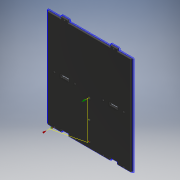
# Autodesk Inventor part: BA04
Saved by Autodesk Inventor 2017 (Build 210142000, 142)
## iProperties
Created: 2019-05-22
Part Number: BA04
Material: Polyethylene, High Density
Document SubType Name: Modeling
Designer: Dell
Density: 0.952 g/cm^3
Appearance: Smooth - Black
Mass: 627.857 g
Surface Area: 2193.54 cm^2
Volume: 659.513 cm^3
Author: Dell
Autodesk Inventor part; units mm, degrees
ref_plane "YZ Plane" through (0, 0, 0) normal (1, 0, 0) x (0, 1, 0)
ref_plane "XZ Plane" through (0, 0, 0) normal (0, 1, 0) x (-1, 0, 0)
ref_plane "XY Plane" through (0, 0, 0) normal (0, 0, 1) x (1, 0, 0)
sketch "Sketch1" plane through (0, 0, 0) normal (0, 0, 1) x (1, 0, 0)
  line L0 (0, 0) -> (303.5592, 0)
  line L1 (303.5592, 0) -> (455.3388, -262.89) construction
  line L2 (455.3388, -262.89) -> (404.5388, -350.8782)
  line L3 (404.5388, -350.8782) -> (-50.8, -87.9882) construction
  line L4 (-50.8, -87.9882) -> (0, 0) construction
  line L5 (0, 0) -> (3.6662, -6.35)
  line L6 (3.6662, -6.35) -> (299.8931, -6.35)
  line L7 (299.8931, -6.35) -> (303.5592, 0)
  dimension "d0" = 525.78
  dimension "d1" = 101.6
  dimension "d2" = 120
  dimension "d3" = 6.35
  dimension "d4" = 60
  dimension "d5" = 60
  constraints: 16 end point, 2 equal length, 2 horizontal, 2 perpendicular
  measures "d0" distance of L2.end L3.end
  measures "d1" distance of L3.end L0.start
  measures "d2" angle of L0 L4
  measures "d3" distance between parallel lines of L0 L6
  measures "d4" angle of L0 L5
  measures "d5" angle of L0 L7
extrude "Extrusion1" add sketch "Sketch1" along normal blind 349.25
sketch "Sketch2" plane through (3.6662, -6.35, 0) normal (0, -1, 0) x (1, 0, 0)
  line L0 (299.8931, 349.25) -> (-3.6662, 349.25) projected
  line L1 (47.1338, 349.25) -> (72.5338, 349.25)
  line L2 (72.5338, 349.25) -> (72.5338, 355.6)
  line L3 (72.5338, 355.6) -> (47.1338, 355.6)
  line L4 (47.1338, 355.6) -> (47.1338, 349.25)
  line L5 (223.6931, 349.25) -> (249.0931, 349.25)
  line L6 (249.0931, 349.25) -> (249.0931, 355.6)
  line L7 (249.0931, 355.6) -> (223.6931, 355.6)
  line L8 (223.6931, 355.6) -> (223.6931, 349.25)
  line L9 (-3.6662, 0) -> (-3.6662, 349.25) projected
  line L10 (299.8931, 0) -> (299.8931, 349.25) projected
  circle A0 centre (59.8338, 352.425) radius 2.25
  circle A1 centre (236.3931, 352.425) radius 2.25
  point P0 (59.8338, 355.6)
  point P1 (236.3931, 355.6)
  point P2 (72.5338, 352.425)
  point P3 (249.0931, 352.425)
  dimension "d8" = 25.4
  dimension "d9" = 6.35
  dimension "d10" = 25.4
  dimension "d11" = 6.35
  dimension "d12" = 50.8
  dimension "d13" = 50.8
  dimension "d16" = 4.5
  dimension "d17" = 4.5
  constraints: 16 end point, 4 midpoint, 4 parallel, 2 centre point, 2 horizontal, 2 horizontal alignment, 2 perpendicular, 2 point on line, 2 vertical alignment
  measures "d8" distance of L3.end L2.end
  measures "d9" distance of L2.end L1.end
  measures "d10" distance of L7.end L6.end
  measures "d11" distance of L6.end L5.end
  measures "d12" distance between parallel lines of L9 L4
  measures "d13" distance between parallel lines of L10 L6
  measures "d16" diameter of A0
  measures "d17" diameter of A1
extrude "Extrusion2" add sketch "Sketch2" against normal blind 6.35
ref_plane "Work Plane1" through (0, 0, 298.45) normal (0, 0, 1) x (1, 0, 0)
sketch "Sketch3" plane through (0, 0, 298.45) normal (0, 0, 1) x (1, 0, 0)
  line L0 (0, 0) -> (303.5592, 0) projected
  line L1 (0, 0) -> (0, -6.35)
  line L2 (299.8931, -6.35) -> (3.6662, -6.35) projected
  line L3 (0, -6.35) -> (3.6662, -6.35)
  line L4 (3.6662, -6.35) -> (0, 0) projected
  constraints: 4 end point, 1 perpendicular, 1 vertical
extrude "Extrusion3" [suppressed]
ref_plane "Work Plane2" through (0, 0, 50.8) normal (0, 0, -1) x (-1, 0, 0)
sketch "Sketch4" plane through (0, 0, 50.8) normal (0, 0, -1) x (-1, 0, 0)
  line L0 (0, -12.7) -> (0, 0) projected
  line L1 (-7.3323, -12.7) -> (0, 0) projected
  line L2 (-7.3323, -12.7) -> (0, -12.7) projected
extrude "Extrusion4" [suppressed]
ref_plane "Work Plane3" through (0, 0, 174.625) normal (0, 0, -1) x (-1, 0, 0)
sketch "Sketch5" plane through (0, 0, 174.625) normal (0, 0, -1) x (-1, 0, 0)
  line L0 (0, 0) -> (0, -12.7) projected
  line L1 (0, -12.7) -> (-7.3323, -12.7) projected
  line L2 (0, 0) -> (-7.3323, -12.7) projected
extrude "Extrusion5" [suppressed]
ref_plane "Work Plane4" through (151.7796, -6.35, 349.25) normal (-1, 0, 0) x (0, 0, 1)
mirror "Mirror1" [suppressed]
sketch "Sketch6" plane through (296.2269, -12.7, 292.1) normal (0, 0, 1) x (1, 0, 0)
  line L0 (0, 0) -> (7.3323, 12.7) projected
  line L1 (7.3323, 0) -> (0, 0) projected
  line L2 (7.3323, 12.7) -> (7.3323, 0) projected
  line L3 (7.3323, 12.7) -> (7.3323, 0) projected
  line L4 (0, 0) -> (7.3323, 12.7) projected
  line L5 (7.3323, 0) -> (0, 0) projected
  line L6 (-296.2269, 12.7) -> (-296.2269, 0) projected
  line L7 (-296.2269, 0) -> (-288.8945, 0) projected
  line L8 (-296.2269, 12.7) -> (-288.8945, 0) projected
  line L9 (-296.2269, 0) -> (-296.2269, 12.7) projected
  line L10 (-296.2269, 12.7) -> (-274.2298, 0) construction
  line L11 (0, 0) -> (-288.8945, 0) projected
  line L12 (-285.2269, 6.3491) -> (-285.2269, 0)
  line L13 (-288.8945, 0) -> (-296.2269, 0) projected
  line L14 (-285.2269, 0) -> (-296.2269, 0)
  line L15 (-144.4473, 0) -> (-144.4473, -42.8761)
  line L16 (7.3323, 12.7) -> (7.3323, 0)
  line L17 (7.3323, 0) -> (0, 0)
  line L18 (7.3323, 12.7) -> (0, 0)
  line L19 (7.3323, 0) -> (7.3323, 12.7)
  line L20 (7.3323, 12.7) -> (-14.6647, 0) construction
  line L21 (-3.6677, 6.3491) -> (-3.6677, 0)
  line L22 (0, 0) -> (7.3323, 0)
  line L23 (-3.6677, 0) -> (7.3323, 0)
  line L24 (-288.8945, 0) -> (-296.2269, 12.7) projected
  line L25 (-285.2269, 6.3491) -> (-296.2269, 12.7)
  line L26 (7.3323, 12.7) -> (0, 0) projected
  line L27 (7.3323, 12.7) -> (-3.6677, 6.3491)
  line L28 (0, 0) -> (7.3323, 12.7)
  line L29 (0, 0) -> (-3.6677, 0)
  line L30 (7.3323, 0) -> (7.3323, 12.7) projected
  line L31 (-3.6677, 0) -> (7.3323, 0)
  dimension "d26" = 60
  dimension "d27" = 11
  constraints: 34 end point, 5 symmetric about line, 3 point on line, 2 collinear, 2 horizontal, 1 midpoint, 1 perpendicular, 1 vertical
  measures "d26" angle of L6 L10
  measures "d27" distance between parallel lines of L6 L12
extrude "Extrusion6" [suppressed]
sketch "Sketch7" plane through (0, 0, 184.15) normal (0, 0, 1) x (1, 0, 0)
  line L0 (7.3323, -12.7) -> (0, 0) projected
  line L1 (11, -12.7) -> (7.3323, -12.7) projected
  line L2 (11, -6.3509) -> (11, -12.7) projected
  line L3 (0, 0) -> (11, -6.3509) projected
  line L4 (303.5592, 0) -> (296.2269, -12.7) projected
  line L5 (292.5592, -6.3509) -> (303.5592, 0) projected
  line L6 (292.5592, -12.7) -> (292.5592, -6.3509) projected
  line L7 (296.2269, -12.7) -> (292.5592, -12.7) projected
  line L8 (303.5592, 0) -> (303.5592, -12.7) projected
  line L9 (296.2269, -12.7) -> (303.5592, 0) projected
  line L10 (303.5592, -12.7) -> (296.2269, -12.7) projected
  line L11 (0, 0) -> (0, -12.7) projected
  line L12 (0, -12.7) -> (7.3323, -12.7) projected
  line L13 (0, 0) -> (7.3323, -12.7) projected
extrude "Extrusion7" [suppressed]
sketch "Sketch8" plane through (0, 0, 76.2) normal (0, 0, 1) x (1, 0, 0)
  line L0 (0, 0) -> (0, -12.7) projected
  line L1 (0, -12.7) -> (7.3323, -12.7) projected
  line L2 (0, 0) -> (7.3323, -12.7) projected
  line L3 (7.3323, -12.7) -> (0, 0) projected
  line L4 (11, -12.7) -> (7.3323, -12.7) projected
  line L5 (11, -6.3509) -> (11, -12.7) projected
  line L6 (0, 0) -> (11, -6.3509) projected
  line L7 (303.5592, 0) -> (296.2269, -12.7) projected
  line L8 (292.5592, -6.3509) -> (303.5592, 0) projected
  line L9 (292.5592, -12.7) -> (292.5592, -6.3509) projected
  line L10 (296.2269, -12.7) -> (292.5592, -12.7) projected
  line L11 (303.5592, 0) -> (303.5592, -12.7) projected
  line L12 (296.2269, -12.7) -> (303.5592, 0) projected
  line L13 (303.5592, -12.7) -> (296.2269, -12.7) projected
extrude "Extrusion8" [suppressed]
sketch "Sketch9" plane through (0, 0, 0) normal (0, 0, -1) x (-1, 0, 0)
  line L0 (-251.9796, -6.35) -> (-251.9796, 0)
  line L1 (-251.9796, 0) -> (-226.5796, 0)
  line L2 (-226.5796, 0) -> (-226.5796, -6.35)
  line L3 (-226.5796, -6.35) -> (-251.9796, -6.35)
  line L4 (-76.9796, -6.35) -> (-76.9796, 0)
  line L5 (-76.9796, 0) -> (-51.5796, 0)
  line L6 (-51.5796, 0) -> (-51.5796, -6.35)
  line L7 (-51.5796, -6.35) -> (-76.9796, -6.35)
  line L8 (-239.2796, 0) -> (-64.2796, 0) construction
  circle A0 centre (-239.2796, -3.175) radius 2.25
  circle A1 centre (-64.2796, -3.175) radius 2.25
  line L9 (-239.2796, -3.175) -> (-239.2796, 0) construction
  line L10 (-239.2796, -3.175) -> (-226.5796, -3.175) construction
  line L11 (-76.9796, -3.175) -> (-64.2796, -3.175) construction
  line L12 (-64.2796, -3.175) -> (-64.2796, 0) construction
  line L13 (0, 0) -> (-303.5592, 0) projected
  point P0 (-151.7796, 0)
  dimension "d34" = 25.4
  dimension "d35" = 6.35
  dimension "d36" = 6.35
  dimension "d37" = 25.4
  dimension "d38" = 175
  dimension "d39" = 4.5
  dimension "d40" = 4.5
  constraints: 26 end point, 6 midpoint, 6 perpendicular, 4 parallel, 4 point on line, 2 centre point
  measures "d34" distance of L4.end L5.end
  measures "d35" distance of L5.end L7.start
  measures "d36" distance of L0.start L1.start
  measures "d37" distance of L1.start L2.start
  measures "d38" distance of L8.start L12.end
  measures "d39" diameter of A0
  measures "d40" diameter of A1
extrude "Extrusion9" cut sketch "Sketch9" against normal blind 6.35 contours L0 L1 L2 L3 | L4 L5 L6 L7 | A0 | A1
sketch "Sketch10" plane through (227.3592, -6.35, 355.6) normal (0, -1, 0) x (1, 0, 0)
  line L0 (-175.7796, -184.625) -> (-150.3796, -184.625)
  line L1 (-150.3796, -184.625) -> (-150.3796, -178.275)
  line L2 (-150.3796, -178.275) -> (-175.7796, -178.275)
  line L3 (-175.7796, -178.275) -> (-175.7796, -184.625)
  line L4 (-0.7796, -184.625) -> (24.6204, -184.625)
  line L5 (24.6204, -184.625) -> (24.6204, -178.275)
  line L6 (24.6204, -178.275) -> (-0.7796, -178.275)
  line L7 (-0.7796, -178.275) -> (-0.7796, -184.625)
  line L8 (-175.7796, -349.25) -> (-150.3796, -349.25) projected
  line L9 (-0.7796, -349.25) -> (24.6204, -349.25) projected
  line L10 (76.2, -6.35) -> (-227.3592, -6.35) projected
  point P0 (-227.3592, -355.6)
  point P1 (-163.0796, -184.625)
  point P2 (-163.0796, -349.25)
  point P3 (11.9204, -184.625)
  point P4 (11.9204, -349.25)
  point P5 (-176.5592, -6.35)
  dimension "d44" = 25.4
  dimension "d45" = 6.35
  dimension "d46" = 25.4
  dimension "d47" = 6.35
  dimension "d90" = 171.925
  constraints: 16 end point, 4 midpoint, 4 parallel, 2 horizontal, 2 perpendicular, 2 vertical alignment, 1 horizontal alignment
  measures "d44" distance of L2.end L1.end
  measures "d45" distance of L1.end L0.end
  measures "d46" distance of L6.end L5.end
  measures "d47" distance of L5.end L4.end
  measures "d90" distance between parallel lines of L10 L2
extrude "Extrusion10" cut sketch "Sketch10" against normal through all
sketch "Sketch11" plane through (227.3592, -6.35, 355.6) normal (0, -1, 0) x (1, 0, 0)
  line L0 (-150.3796, -355.6) -> (-0.7796, -355.6) construction
  line L1 (-100.9796, -355.6) -> (-50.1796, -355.6) construction
  line L2 (-50.1796, -355.6) -> (-50.1796, -178.275) construction
  line L3 (-50.1796, -178.275) -> (-100.9796, -178.275) construction
  line L4 (-100.9796, -178.275) -> (-100.9796, -355.6) construction
  circle A0 centre (-75.5796, -267.89) radius 4
  circle A1 centre (-75.5796, -200.18) radius 4
  circle A2 centre (-75.5796, -335.6) radius 4
  line L5 (-0.7796, -355.6) -> (-150.3796, -355.6) projected
  circle A3 centre (-199.7363, -181.45) radius 2.25
  circle A4 centre (-199.7363, -352.425) radius 2.25
  circle A5 centre (48.5771, -352.425) radius 2.25
  circle A6 centre (48.5771, -181.45) radius 2.25
  line L6 (-175.7796, -355.6) -> (-223.6931, -355.6) projected
  line L7 (72.5338, -355.6) -> (24.6204, -355.6) projected
  line L8 (-175.7796, -184.625) -> (-175.7796, -178.275) projected
  line L9 (-175.7796, -355.6) -> (-175.7796, -349.25) projected
  line L10 (24.6204, -349.25) -> (24.6204, -355.6) projected
  line L11 (24.6204, -178.275) -> (24.6204, -184.625) projected
  circle A7 centre (-126.3796, -181.45) radius 2.25
  circle A8 centre (-126.3796, -352.425) radius 2.25
  circle A9 centre (-24.7796, -352.425) radius 2.25
  circle A10 centre (-24.7796, -181.45) radius 2.25
  point P0 (-227.3592, -355.6)
  point P1 (-150.3796, -178.275)
  point P2 (-75.5796, -355.6)
  point P3 (-75.5796, -355.6)
  point P4 (-75.5796, -355.6)
  point P5 (-50.1796, -266.9375)
  point P6 (-199.7363, -355.6)
  point P7 (48.5771, -355.6)
  point P8 (-175.7796, -181.45)
  point P9 (-175.7796, -352.425)
  point P10 (24.6204, -352.425)
  point P11 (24.6204, -181.45)
  point P12 (24.6204, -352.425)
  dimension "d52" = 8
  dimension "d53" = 8
  dimension "d54" = 8
  dimension "d56" = 20
  dimension "d59" = 50.8
  dimension "d60" = 4.5
  dimension "d61" = 4.5
  dimension "d62" = 4.5
  dimension "d63" = 4.5
  dimension "d64" = 4.5
  dimension "d65" = 4.5
  dimension "d66" = 4.5
  dimension "d67" = 4.5
  dimension "d68" = 25.4
  dimension "d69" = 25.4
  dimension "d96" = 67.71
  dimension "d97" = 67.71
  constraints: 11 centre point, 11 midpoint, 9 horizontal alignment, 9 vertical alignment, 8 end point, 2 parallel, 1 coincident, 1 horizontal, 1 perpendicular, 1 point on line
  measures "d52" diameter of A0
  measures "d53" diameter of A1
  measures "d54" diameter of A2
  measures "d56" distance from line of L0 A2.centre
  measures "d59" distance of L2.end L3.end
  measures "d60" diameter of A3
  measures "d61" diameter of A4
  measures "d62" diameter of A5
  measures "d63" diameter of A6
  measures "d64" diameter of A7
  measures "d65" diameter of A8
  measures "d66" diameter of A9
  measures "d67" diameter of A10
  measures "d68" distance from line of L2 A10.centre
  measures "d69" distance from line of A7.centre L4
  measures "d96" distance of A0.centre A1.centre
  measures "d97" distance of A2.centre A0.centre
extrude "Extrusion11" cut sketch "Sketch11" against normal through all
sketch "Sketch12" plane through (227.3592, -6.35, 355.6) normal (0, -1, 0) x (1, 0, 0)
  line L0 (-175.7796, -355.6) -> (-223.6931, -355.6) projected
  line L1 (-177.0496, -355.6) -> (-149.1096, -355.6)
  line L2 (-149.1096, -355.6) -> (-149.1096, -347.98)
  line L3 (-149.1096, -347.98) -> (-177.0496, -347.98)
  line L4 (-177.0496, -347.98) -> (-177.0496, -355.6)
  line L5 (-0.7796, -355.6) -> (-150.3796, -355.6) projected
  line L6 (-2.0496, -355.6) -> (25.8904, -355.6)
  line L7 (25.8904, -355.6) -> (25.8904, -347.98)
  line L8 (25.8904, -347.98) -> (-2.0496, -347.98)
  line L9 (-2.0496, -347.98) -> (-2.0496, -355.6)
  line L10 (-177.0496, -177.005) -> (-149.1096, -177.005)
  line L11 (-149.1096, -177.005) -> (-149.1096, -185.895)
  line L12 (-149.1096, -185.895) -> (-177.0496, -185.895)
  line L13 (-177.0496, -185.895) -> (-177.0496, -177.005)
  line L14 (-2.0496, -177.005) -> (25.8904, -177.005)
  line L15 (25.8904, -177.005) -> (25.8904, -185.895)
  line L16 (25.8904, -185.895) -> (-2.0496, -185.895)
  line L17 (-2.0496, -185.895) -> (-2.0496, -177.005)
  line L18 (-150.3796, -178.275) -> (-150.3796, -184.625) projected
  line L19 (-0.7796, -184.625) -> (-0.7796, -178.275) projected
  line L20 (-175.7796, -178.275) -> (-150.3796, -178.275) projected
  line L21 (-0.7796, -178.275) -> (24.6204, -178.275) projected
  line L22 (-0.7796, -349.25) -> (24.6204, -349.25) projected
  line L23 (-175.7796, -349.25) -> (-150.3796, -349.25) projected
  circle A0 centre (-178.8043, -4.1049) radius 3.175
  circle A1 centre (-148.9142, -4.1049) radius 3.175
  circle A2 centre (-2.2451, -4.1049) radius 3.175
  circle A3 centre (27.6451, -4.1049) radius 3.175
  line L24 (-176.5592, -6.35) -> (-178.8043, -4.1049)
  line L25 (-223.6931, -6.35) -> (-176.5592, -6.35) projected
  point P0 (-227.3592, -355.6)
  point P1 (-150.3796, -181.45)
  point P2 (-149.1096, -181.45)
  point P3 (-0.7796, -181.45)
  point P4 (-2.0496, -181.45)
  point P5 (-163.0796, -178.275)
  point P6 (-163.0796, -177.005)
  point P7 (11.9204, -178.275)
  point P8 (11.9204, -177.005)
  point P9 (11.9204, -349.25)
  point P10 (11.9204, -347.98)
  point P11 (-163.0796, -349.25)
  point P12 (-163.0796, -347.98)
  point P13 (-151.1592, -6.35)
  point P14 (0, -6.35)
  point P15 (25.4, -6.35)
  dimension "d74" = 6.35
  dimension "d75" = 6.35
  dimension "d76" = 6.35
  dimension "d77" = 6.35
  dimension "d70" = 1.27
  dimension "d71" = 1.27
  dimension "d72" = 1.27
  dimension "d73" = 1.27
  dimension "d89" = 45
  constraints: 34 end point, 12 midpoint, 8 parallel, 7 horizontal alignment, 5 vertical alignment, 4 horizontal, 4 perpendicular, 3 point on line, 12 other
  measures "d70" distance between parallel lines of L10 L20
  measures "d71" distance between parallel lines of L17 L19
  measures "d72" distance between parallel lines of L11 L18
  measures "d73" distance between parallel lines of L3 L23
  measures "d89" angle of L25 L24
extrude "Extrusion12" cut sketch "Sketch12" against normal through all
sketch "Sketch13" plane through (227.3592, -6.35, 355.6) normal (0, -1, 0) x (1, 0, 0)
  line L0 (-176.5592, 0) -> (-151.1592, 0)
  line L1 (-151.1592, 0) -> (-151.1592, 1.27)
  line L2 (-151.1592, 1.27) -> (-176.5592, 1.27)
  line L3 (-176.5592, 1.27) -> (-176.5592, 0)
  line L4 (25.4, 0) -> (0, 0)
  line L5 (0, 0) -> (0, 1.27)
  line L6 (0, 1.27) -> (25.4, 1.27)
  line L7 (25.4, 1.27) -> (25.4, 0)
  point P0 (-227.3592, -355.6)
  point P1 (-151.1592, 0)
  dimension "d80" = 1.27
  constraints: 16 end point, 4 parallel, 2 coincident, 2 horizontal, 2 perpendicular, 1 horizontal alignment
  measures "d80" distance of L2.end L0.start
extrude "Extrusion13" add sketch "Sketch13" against normal up to surface (6.35 mm away) from surface at 0
sketch "Sketch14" plane through (299.8931, -6.35, 0) normal (0, -1, 0) x (1, 0, 0)
  line L0 (-47.1338, 356.87) -> (-72.5338, 356.87) projected
  line L1 (-47.1338, 356.87) -> (-47.7688, 356.87)
  line L2 (-47.7688, 356.87) -> (-47.7688, 352.8314)
  line L3 (-47.7688, 352.8314) -> (-47.1338, 352.8314)
  line L4 (-47.1338, 352.8314) -> (-47.1338, 356.87)
  arc A0 (-77.024, 349.25) -> (-72.5338, 353.7401) centre (-74.7789, 351.4951) ccw projected
  line L5 (-72.5338, 356.87) -> (-71.8988, 356.87)
  line L6 (-71.8988, 356.87) -> (-71.8988, 352.8314)
  line L7 (-71.8988, 352.8314) -> (-72.5338, 352.8314)
  line L8 (-72.5338, 352.8314) -> (-72.5338, 356.87)
  arc A1 (-223.6931, 353.7401) -> (-219.2029, 349.25) centre (-221.448, 351.4951) ccw projected
  line L9 (-223.6931, 356.87) -> (-224.3281, 356.87)
  line L10 (-224.3281, 356.87) -> (-224.3281, 352.8314)
  line L11 (-224.3281, 352.8314) -> (-223.6931, 352.8314)
  line L12 (-223.6931, 352.8314) -> (-223.6931, 356.87)
  line L13 (-249.0931, 356.87) -> (-249.0931, 353.7401) projected
  line L14 (-249.0931, 356.87) -> (-248.4581, 356.87)
  line L15 (-248.4581, 356.87) -> (-248.4581, 352.8314)
  line L16 (-248.4581, 352.8314) -> (-249.0931, 352.8314)
  line L17 (-249.0931, 352.8314) -> (-249.0931, 356.87)
  point P0 (-299.8931, 0)
  dimension "d91" = 0.635
  dimension "d92" = 0.635
  dimension "d93" = 0.635
  constraints: 32 end point, 8 parallel, 4 horizontal, 4 perpendicular, 3 point on line, 2 point on circle
  measures "d91" distance between parallel lines of L13 L15
  measures "d92" distance between parallel lines of L12 L10
  measures "d93" distance between parallel lines of L4 L2
extrude "Extrusion14" cut sketch "Sketch14" against normal through all
sketch "Sketch16" plane through (3.6662, -6.35, 0) normal (0, -1, 0) x (1, 0, 0)
  line L0 (71.8988, 352.8314) -> (71.8988, 356.87) construction
  line L1 (47.7688, 356.87) -> (71.8988, 356.87) construction
  line L2 (47.7688, 356.87) -> (47.7688, 352.8314) construction
  arc A0 (42.6437, 349.25) -> (47.7688, 352.8314) centre (44.8888, 351.4951) ccw construction
  line L3 (0, 349.25) -> (42.6437, 349.25) construction
  line L4 (0, 0) -> (0, 349.25) construction
  line L5 (46.6434, 0) -> (0, 0) construction
  line L6 (46.6434, 0) -> (46.6434, 7.62) construction
  line L7 (46.6434, 7.62) -> (74.5834, 7.62) construction
  line L8 (74.5834, 7.62) -> (74.5834, 0) construction
  line L9 (221.6434, 0) -> (74.5834, 0) construction
  line L10 (221.6434, 0) -> (221.6434, 7.62) construction
  line L11 (221.6434, 7.62) -> (249.5834, 7.62) construction
  line L12 (249.5834, 7.62) -> (249.5834, 0) construction
  line L13 (296.2269, 0) -> (249.5834, 0) construction
  line L14 (296.2269, 0) -> (296.2269, 349.25) construction
  line L15 (253.5832, 349.25) -> (296.2269, 349.25) construction
  arc A1 (248.4581, 352.8314) -> (253.5832, 349.25) centre (251.3381, 351.4951) ccw construction
  line L16 (248.4581, 352.8314) -> (248.4581, 356.87) construction
  line L17 (224.3281, 356.87) -> (248.4581, 356.87) construction
  line L18 (224.3281, 356.87) -> (224.3281, 352.8314) construction
  arc A2 (219.2029, 349.25) -> (224.3281, 352.8314) centre (221.448, 351.4951) ccw construction
  line L19 (77.024, 349.25) -> (219.2029, 349.25) construction
  arc A3 (71.8988, 352.8314) -> (77.024, 349.25) centre (74.7789, 351.4951) ccw construction
  circle A4 centre (59.8338, 352.425) radius 2.25 construction
  circle A5 centre (236.3931, 352.425) radius 2.25 construction
  circle A6 centre (148.1134, 20) radius 4 construction
  circle A7 centre (148.1134, 87.71) radius 4 construction
  circle A8 centre (198.9134, 3.175) radius 2.25 construction
  circle A9 centre (97.3134, 174.15) radius 2.25 construction
  circle A10 centre (272.2702, 3.175) radius 2.25 construction
  circle A11 centre (23.9567, 174.15) radius 2.25 construction
  circle A12 centre (23.9567, 3.175) radius 2.25 construction
  circle A13 centre (272.2702, 174.15) radius 2.25 construction
  circle A14 centre (97.3134, 3.175) radius 2.25 construction
  circle A15 centre (198.9134, 174.15) radius 2.25 construction
  circle A16 centre (148.1134, 155.42) radius 4 construction
  line L20 (221.6434, 169.705) -> (221.6434, 178.595) construction
  line L21 (221.6434, 178.595) -> (249.5834, 178.595) construction
  line L22 (249.5834, 178.595) -> (249.5834, 169.705) construction
  line L23 (249.5834, 169.705) -> (221.6434, 169.705) construction
  line L24 (46.6434, 169.705) -> (46.6434, 178.595) construction
  line L25 (46.6434, 178.595) -> (74.5834, 178.595) construction
  line L26 (74.5834, 178.595) -> (74.5834, 169.705) construction
  line L27 (74.5834, 169.705) -> (46.6434, 169.705) construction
  line L28 (222.083, 351.4951) -> (222.083, 359.1151) construction
  line L29 (222.083, 359.1151) -> (250.7031, 359.1151) construction
  line L30 (250.7031, 359.1151) -> (250.7031, 351.4951) construction
  line L31 (250.7031, 351.4951) -> (298.4719, 351.4951) construction
  line L32 (298.4719, 351.4951) -> (298.4719, -2.2451) construction
  line L33 (298.4719, -2.2451) -> (247.3384, -2.2451) construction
  line L34 (247.3384, -2.2451) -> (247.3384, 5.3749) construction
  line L35 (247.3384, 5.3749) -> (223.8885, 5.3749) construction
  line L36 (223.8885, 5.3749) -> (223.8885, -2.2451) construction
  line L37 (223.8885, -2.2451) -> (72.3384, -2.2451) construction
  line L38 (72.3384, -2.2451) -> (72.3384, 5.3749) construction
  line L39 (72.3384, 5.3749) -> (48.8885, 5.3749) construction
  line L40 (48.8885, 5.3749) -> (48.8885, -2.2451) construction
  line L41 (48.8885, -2.2451) -> (-2.2451, -2.2451) construction
  line L42 (-2.2451, -2.2451) -> (-2.2451, 351.4951) construction
  line L43 (-2.2451, 351.4951) -> (45.5238, 351.4951) construction
  line L44 (45.5238, 351.4951) -> (45.5238, 359.1151) construction
  line L45 (45.5238, 359.1151) -> (74.1439, 359.1151) construction
  line L46 (74.1439, 359.1151) -> (74.1439, 351.4951) construction
  line L47 (74.1439, 351.4951) -> (222.083, 351.4951) construction
  line L48 (72.3384, 176.3499) -> (48.8885, 176.3499) construction
  line L49 (48.8885, 176.3499) -> (48.8885, 171.9501) construction
  line L50 (48.8885, 171.9501) -> (72.3384, 171.9501) construction
  line L51 (72.3384, 171.9501) -> (72.3384, 176.3499) construction
  line L52 (247.3384, 176.3499) -> (223.8885, 176.3499) construction
  line L53 (223.8885, 176.3499) -> (223.8885, 171.9501) construction
  line L54 (223.8885, 171.9501) -> (247.3384, 171.9501) construction
  line L55 (247.3384, 171.9501) -> (247.3384, 176.3499) construction
  circle A17 centre (48.8885, 5.3749) radius 3.175
  circle A18 centre (72.3384, 5.3749) radius 3.175
  line L56 (221.6434, 7.62) -> (249.5834, 7.62) projected
  circle A19 centre (223.8885, 5.3749) radius 3.175
  circle A20 centre (247.3384, 5.3749) radius 3.175
  line L57 (221.6434, 178.595) -> (249.5834, 178.595) projected
  circle A21 centre (247.3384, 176.3499) radius 3.175
  circle A22 centre (247.3384, 171.9501) radius 3.175
  line L58 (249.5834, 169.705) -> (221.6434, 169.705) projected
  circle A23 centre (223.8885, 171.9501) radius 3.175
  circle A24 centre (223.8885, 176.3499) radius 3.175
  circle A25 centre (72.3384, 176.3499) radius 3.175
  line L59 (74.5834, 169.705) -> (74.5834, 178.595) projected
  circle A26 centre (72.3384, 171.9501) radius 3.175
  line L60 (74.5834, 169.705) -> (46.6434, 169.705) projected
  circle A27 centre (48.8885, 171.9501) radius 3.175
  line L61 (74.5834, 178.595) -> (46.6434, 178.595) projected
  circle A28 centre (48.8885, 176.3499) radius 3.175
  point P0 (-3.6662, 0)
  dimension "d98" = 6.35
  dimension "d99" = 6.35
  dimension "d100" = 6.35
  constraints: 56 end point, 12 coincident, 61 other
extrude "Extrusion15" cut sketch "Sketch16" against normal through all contours A17 | A18 | A19 L56 | L56 A19 | A20 L56 | L56 A20 | A24 L57 | L57 A24 A23 | A24 A23 L58 | A23 A24 | A21 L57 | L57 A21 A22 | L58 A23 | A22 A21 | A21 A22 L58 | L58 A22 | A25 A26 L59 | L61 A25 | L59 A26 A25 L61 | A26 L59 A25 | A25 L59 A26 | L59 A25 A26 | L59 L60 A26 A25 | A28 A27 L61 | L61 A28 | A26 L60 | A27 L60 | L60 A27 A28 | A27 A28
equation "\"d3\" = Panel_Thickness"
equation "\"d9\" = Panel_Thickness"
equation "\"d11\" = Panel_Thickness"
equation "\"d14\" = Panel_Thickness"
equation "\"d35\" = Panel_Thickness"
equation "\"d36\" = Panel_Thickness"
equation "\"d42\" = Panel_Thickness"
equation "\"d45\" = Panel_Thickness"
equation "\"d47\" = Panel_Thickness"
equation "\"d74\" = Tool_Dia"
equation "\"d75\" = Tool_Dia"
equation "\"d76\" = Tool_Dia"
equation "\"d77\" = Tool_Dia"
equation "\"d70\" = Fit_Tolerance"
equation "\"d71\" = Fit_Tolerance"
equation "\"d72\" = Fit_Tolerance"
equation "\"d73\" = Fit_Tolerance"
equation "\"d80\" = Fit_Tolerance"
equation "\"d91\" = 0.5 * Fit_Tolerance"
equation "\"d92\" = 0.5 * Fit_Tolerance"
equation "\"d93\" = 0.5 * Fit_Tolerance"
equation "\"d98\" = Tool_Dia"
equation "\"d99\" = Tool_Dia"
equation "\"d100\" = Tool_Dia"
equation "\"Panel_Thickness\" = 6.35"
equation "\"Fit_Tolerance\" = 1.27"
equation "\"Tool_Dia\" = 6.35"
body "Solid1"
